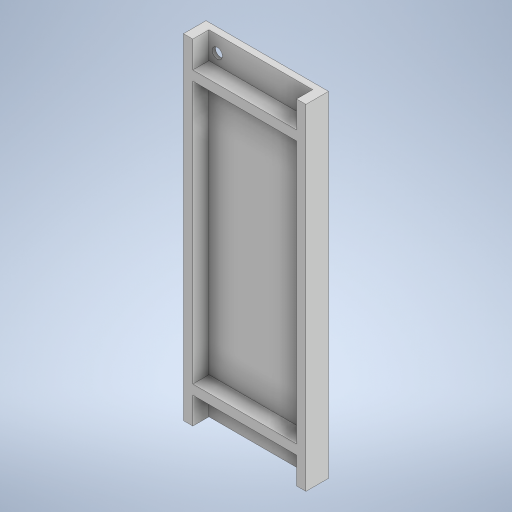
# Autodesk Inventor part: robot-arm-frame
Saved by Autodesk Inventor 2024.3 (Build 283343000, 343)
## iProperties
Created: 2024-11-10
Part Number: robot-arm-frame
Material: 一般
Document SubType Name: Modeling
Designer: azara
Density: 1 g/cm^3
Appearance: 既定
Author: azara
Autodesk Inventor part; units mm, degrees
ref_plane "YZ Plane" through (0, 0, 0) normal (1, 0, 0) x (0, 1, 0)
ref_plane "XZ Plane" through (0, 0, 0) normal (0, 1, 0) x (-1, 0, 0)
ref_plane "XY Plane" through (0, 0, 0) normal (0, 0, 1) x (1, 0, 0)
sketch "スケッチ1" plane through (0, 0, 0) normal (0, 0, 1) x (1, 0, 0)
  line L0 (0, 0) -> (38, 0)
  line L1 (38, 0) -> (38, 104)
  line L2 (38, 104) -> (0, 104)
  line L3 (0, 104) -> (0, 0)
  dimension "d0" = 38
  dimension "d1" = 104
  constraints: 8 end point, 2 parallel, 1 horizontal, 1 perpendicular
  measures "d0" distance of L0.start L0.end
  measures "d1" distance of L0.end L1.end
extrude "押し出し1" add sketch "スケッチ1" along normal blind 2
sketch "スケッチ2" plane through (0, 0, 2) normal (0, 0, 1) x (1, 0, 0)
  line L0 (38, 104) -> (0, 104) projected
  line L1 (0, 0) -> (38, 0)
  line L2 (38, 0) -> (38, 104)
  line L3 (38, 104) -> (0, 104)
  line L4 (0, 104) -> (0, 0)
  line L5 (2.9, 0) -> (35.1, 0)
  line L6 (35.1, 0) -> (35.1, 104)
  line L7 (35.1, 104) -> (2.9, 104)
  line L8 (2.9, 104) -> (2.9, 0)
  point P0 (2.9, 0)
  dimension "d4" = 2.9
  dimension "d5" = 2.9
  dimension "d6" = 0
  dimension "d7" = 0
  constraints: 16 end point, 4 parallel, 2 horizontal, 2 perpendicular
  measures "d4" distance between parallel lines of L2 L6
  measures "d5" distance between parallel lines of L4 L8
  measures "d6" distance between parallel lines of L1 L5
  measures "d7" distance between parallel lines of L7 L0
extrude "押し出し2" add sketch "スケッチ2" along normal blind 5 contours L2 L1 L6 L0 | L8 L1 L4 L0
sketch "スケッチ3" plane through (0, 0, 0) normal (0, 0, -1) x (-1, 0, 0)
  line L0 (-38, 104) -> (0, 104) projected
  line L1 (0, 0) -> (-38, 0) projected
  line L2 (-35.1, 0) -> (-35.1, 104) projected
  line L3 (-2.9, 104) -> (-2.9, 0) projected
  point P0 (-32.5, 99)
  point P1 (-5.5, 99)
  point P2 (-5.5, 5)
  point P3 (-32.5, 5)
  dimension "d10" = 5
  dimension "d11" = 5
  dimension "d12" = 5
  dimension "d13" = 5
  dimension "d14" = 27
  dimension "d15" = 2.6
  dimension "d16" = 27
  dimension "d17" = 2.6
  measures "d10" distance from line of L0 point (-32.5, 99)
  measures "d11" distance from line of L0 point (-5.5, 99)
  measures "d12" distance from line of L1 point (-5.5, 5)
  measures "d13" distance from line of L1 point (-32.5, 5)
  measures "d14" distance of point (-5.5, 5) point (-32.5, 5)
  measures "d15" distance from line of L2 point (-32.5, 5)
  measures "d16" distance of point (-5.5, 99) point (-32.5, 99)
  measures "d17" distance from line of L2 point (-32.5, 99)
hole "穴1" at (32.5, 99, 0) at (5.5, 99, 0) at (5.5, 5, 0) at (32.5, 5, 0) direction (0, 0, 1) diameter 3.2 end through all
sketch "スケッチ4" plane through (0, 0, 0) normal (0, 0, -1) x (-1, 0, 0)
  circle A0 centre (-32.5, 99) radius 1.6 projected
  circle A1 centre (-5.5, 99) radius 1.6 projected
  circle A2 centre (-32.5, 5) radius 1.6 projected
  line L0 (0, 104) -> (0, 0) projected
  line L1 (0, 0) -> (-38, 0) projected
  circle A3 centre (-32.5, 99) radius 4
  circle A4 centre (-5.5, 99) radius 4
  circle A5 centre (-32.5, 5) radius 4
  circle A6 centre (-5.5, 5) radius 1.6 projected
  circle A7 centre (-5.5, 5) radius 4
  point P0 (-5.5, 15)
  dimension "d25" = 5.5
  dimension "d26" = 15
  dimension "d27" = 8
  dimension "d28" = 8
  dimension "d29" = 8
  dimension "d30" = 8
  constraints: 7 coincident, 4 centre point
  measures "d25" distance from line of L0 point (-5.5, 15)
  measures "d26" distance from line of L1 point (-5.5, 15)
  measures "d27" diameter of A3
  measures "d28" diameter of A4
  measures "d29" diameter of A5
  measures "d30" diameter of A7
extrude "押し出し3" cut sketch "スケッチ4" against normal blind 1
sketch "スケッチ5" plane through (0, 0, 2) normal (0, 0, 1) x (1, 0, 0)
  line L0 (2.9, 104) -> (2.9, 0) projected
  line L1 (35.1, 0) -> (35.1, 104) projected
  line L2 (2.9, 8.3) -> (35.1, 8.3)
  line L3 (35.1, 8.3) -> (35.1, 11.3)
  line L4 (35.1, 11.3) -> (2.9, 11.3)
  line L5 (2.9, 11.3) -> (2.9, 8.3)
  line L6 (2.9, 95.7) -> (35.1, 95.7)
  line L7 (35.1, 95.7) -> (35.1, 92.7)
  line L8 (35.1, 92.7) -> (2.9, 92.7)
  line L9 (2.9, 92.7) -> (2.9, 95.7)
  circle A0 centre (32.5, 5) radius 1.6 projected
  circle A1 centre (5.5, 5) radius 1.6 projected
  circle A2 centre (5.5, 99) radius 1.6 projected
  circle A3 centre (32.5, 99) radius 1.6 projected
  line L10 (2.9, 104) -> (2.9, 0) projected
  line L11 (2.9, 0) -> (35.1, 0) projected
  line L12 (35.1, 0) -> (35.1, 104) projected
  line L13 (35.1, 104) -> (2.9, 104) projected
  point P0 (0, 0)
  point P1 (2.9, 11.3)
  point P2 (2.9, 92.7)
  point P3 (2.9, 95.7)
  dimension "d33" = 3
  dimension "d34" = 3
  dimension "d35" = 3.3
  dimension "d36" = 3.3
  constraints: 16 end point, 4 parallel, 4 point on line, 2 horizontal, 2 perpendicular
  measures "d33" distance between parallel lines of L8 L6
  measures "d34" distance between parallel lines of L2 L4
  measures "d35" distance from line of L2 A1.centre
  measures "d36" distance from line of L6 A2.centre
extrude "押し出し4" add sketch "スケッチ5" along normal blind 5 contours L6 L1 L8 L0 | L4 L1 L2 L0
